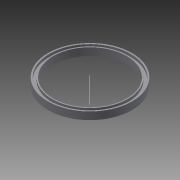
# Autodesk Inventor part: Smaller Cap
Saved by Autodesk Inventor 2015 (Build 190159000, 159)
## iProperties
Created: 2014-07-10
Part Number: Smaller Cap
Material: Generic
Document SubType Name: Modeling
Designer: I Rabey
Density: 1 g/cm^3
Appearance: Default
Author: I Rabey
Autodesk Inventor part; units mm, degrees
ref_plane "YZ Plane" through (0, 0, 0) normal (1, 0, 0) x (0, 1, 0)
ref_plane "XZ Plane" through (0, 0, 0) normal (0, 1, 0) x (-1, 0, 0)
sketch "Sketch1" plane through (0, 0, 0) normal (0, 1, 0) x (-1, 0, 0)
  circle A0 centre (0, 0) radius 28
  circle A1 centre (0, 0) radius 24.5
  dimension "d0" = 56
  dimension "d5" = 49
  constraints: 2 centre point, 2 coincident
  measures "d0" diameter of A0
  measures "d5" diameter of A1
extrude "Extrusion2" add sketch "Sketch1" along normal blind 5
sketch "Sketch3" plane through (0, 5, 0) normal (0, 1, 0) x (1, 0, 0)
  circle A0 centre (0, 0) radius 25.25
  circle A1 centre (0, 0) radius 27.05
  dimension "d8" = 50.5
  dimension "d9" = 54.1
  constraints: 2 centre point, 2 coincident
  measures "d8" diameter of A0
  measures "d9" diameter of A1
extrude "Extrusion3" cut sketch "Sketch3" against normal blind 1.8
ref_plane "Work Plane1" through (0, 4.1, 0) normal (0, -1, 0) x (1, 0, 0)
body "Solid2"
